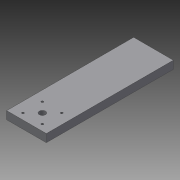
# Autodesk Inventor part: Lead_Screw_Fixture_Base
Saved by Autodesk Inventor 2015 (Build 190159000, 159)
## iProperties
Created: 2014-12-21
Part Number: Lead_Screw_Fixture_Base
Material: Generic
Document SubType Name: Modeling
Designer: Drew
Density: 1 g/cm^3
Appearance: Default
Author: Drew
Autodesk Inventor part; units mm, degrees
ref_plane "YZ Plane" through (0, 0, 0) normal (1, 0, 0) x (0, 1, 0)
ref_plane "XZ Plane" through (0, 0, 0) normal (0, 1, 0) x (-1, 0, 0)
ref_plane "XY Plane" through (0, 0, 0) normal (0, 0, 1) x (1, 0, 0)
sketch "Sketch1" plane through (0, 0, 0) normal (0, 1, 0) x (-1, 0, 0)
  line L0 (-31.75, -101.6) -> (31.75, -101.6)
  line L1 (31.75, -101.6) -> (31.75, 101.6)
  line L2 (31.75, 101.6) -> (-31.75, 101.6)
  line L3 (-31.75, 101.6) -> (-31.75, -101.6)
  line L4 (-31.75, -101.6) -> (31.75, 101.6) construction
  line L5 (31.75, -101.6) -> (-31.75, 101.6) construction
  point P0 (0, 0)
  dimension "d0" = 63.5
  dimension "d1" = 203.2
  constraints: 12 end point, 2 midpoint, 2 parallel, 1 horizontal, 1 perpendicular
  measures "d0" distance of L0.start L0.end
  measures "d1" distance of L0.end L1.end
extrude "Extrusion1" add sketch "Sketch1" along normal blind 12.7
sketch "Sketch2" plane through (0, 12.7, 0) normal (0, 1, 0) x (1, 0, 0)
  line L0 (0, 0) -> (0, -188.6697)
  line L1 (43.5518, -76.2) -> (-58.772, -76.2)
  line L2 (52.9625, 0) -> (-57.3554, 0)
  point P0 (15.494, -91.7)
  point P1 (15.494, -60.7)
  point P2 (-15.494, -91.7)
  point P3 (-15.494, -60.7)
  point P4 (0, -76.2)
  dimension "d6" = 76.2
  dimension "d7" = 31
  dimension "d8" = 30.988
  constraints: 6 end point, 3 horizontal, 3 symmetric about line, 2 point on line, 1 perpendicular, 1 vertical
  measures "d6" distance between parallel lines of L2 L1
  measures "d7" diameter of point (15.494, -91.7) L1
  measures "d8" diameter of point (15.494, -91.7) L0
hole "Hole1" at (15.494, 12.7, 91.7) at (15.494, 12.7, 60.7) at (-15.494, 12.7, 60.7) at (-15.494, 12.7, 91.7) direction (0, -1, 0) diameter 3.5 end through all
sketch "Sketch4" plane through (0, 12.7, 0) normal (0, 1, 0) x (1, 0, 0)
  circle A0 centre (15.494, -60.7) radius 1.75 projected
  circle A1 centre (-15.494, -91.7) radius 1.75 projected
  line L0 (15.494, -60.7) -> (-15.494, -91.7)
  circle A2 centre (-15.494, -60.7) radius 1.75 projected
  circle A3 centre (15.494, -91.7) radius 1.75 projected
  line L1 (-15.494, -60.7) -> (15.494, -91.7)
  point P0 (0, 0)
  point P1 (0, -76.2)
  constraints: 4 end point, 1 midpoint
hole "Hole2" at (0, 12.7, 76.2) direction (0, -1, 0) diameter 10 end through all
body "Solid1"
